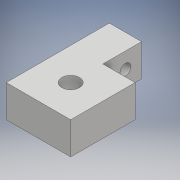
# Autodesk Inventor part: pixymount1
Saved by Autodesk Inventor 2017 (Build 210142000, 142)
## iProperties
Part Number: pixymount1
Material: 一般
Document SubType Name: Modeling
Designer: highs
Density: 1 g/cm^3
Appearance: 既定
Author: highs
## iProperties of the stored document pixymount2_3D プリント.ipt
Part Number: pixymount2_3D プリント
Material: 一般
Document SubType Name: Modeling
Designer: highs
Density: 1 g/cm^3
Appearance: 既定
Author: highs
Autodesk Inventor part; units mm, degrees
ref_plane "YZ Plane" through (0, 0, 0) normal (1, 0, 0) x (0, 1, 0)
ref_plane "XZ Plane" through (0, 0, 0) normal (0, 1, 0) x (-1, 0, 0)
ref_plane "XY Plane" through (0, 0, 0) normal (0, 0, 1) x (1, 0, 0)
sketch "スケッチ4" plane through (0, 0, 0) normal (0, 0, 1) x (1, 0, 0)
  line L0 (0, 0) -> (20, 0)
  line L1 (20, 0) -> (20, 20)
  line L2 (0, 32) -> (0, 0)
  line L3 (0, 32) -> (10, 32)
  line L4 (10, 32) -> (10, 20)
  line L5 (10, 20) -> (20, 20)
  line L6 (10, 0) -> (10, 7.8024) construction
  circle A0 centre (10, 10) radius 2.75
  dimension "d19" = 20
  dimension "d20" = 32
  dimension "d21" = 12
  dimension "d22" = 10
  dimension "d24" = 5.5
  dimension "d25" = 10
  constraints: 14 end point, 3 horizontal, 2 perpendicular, 1 centre point, 1 midpoint, 1 parallel, 1 point on line, 1 vertical
  measures "d19" distance of L0.start L0.end
  measures "d20" distance of L2.start L0.start
  measures "d21" distance of L3.end L4.end
  measures "d22" distance of L2.start L3.end
  measures "d24" diameter of A0
  measures "d25" distance from line of L0 A0.centre
extrude "押し出し4" add sketch "スケッチ4" along normal blind 10
sketch "スケッチ5" plane through (0, 0, 0) normal (-1, 0, 0) x (0, 0, 1)
  line L0 (0, 32) -> (10, 32) projected
  line L1 (5, 32) -> (5, 27) construction
  circle A0 centre (5, 27) radius 1.7
  point P0 (0, 0)
  dimension "d28" = 3.4
  dimension "d29" = 5
  constraints: 2 end point, 1 centre point, 1 coincident, 1 midpoint, 1 vertical
  measures "d28" diameter of A0
  measures "d29" distance from line of L0 A0.centre
extrude "押し出し5" cut sketch "スケッチ5" against normal blind 10
